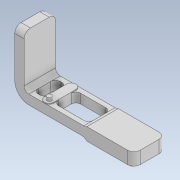
# Autodesk Inventor part: LBody
Saved by Autodesk Inventor 2020 (Build 240168000, 168)
## iProperties
Created: 2020-03-03
Part Number: LBody
Material: Generic
Document SubType Name: Modeling
Designer: Kjell
Density: 1 g/cm^3
Appearance: Default
Author: Kjell
Autodesk Inventor part; units mm, degrees
ref_plane "YZ Plane" through (0, 0, 0) normal (1, 0, 0) x (0, 1, 0)
ref_plane "XZ Plane" through (0, 0, 0) normal (0, 1, 0) x (-1, 0, 0)
ref_plane "XY Plane" through (0, 0, 0) normal (0, 0, 1) x (1, 0, 0)
derived "master_sketch.ipt"
sketch "BottomPlateMainDim" plane through (0, 0, 0) normal (0, 0, 1) x (1, 0, 0)
  circle A0 centre (0, 0) radius 3
  circle A1 centre (-42, -7) radius 1.5
  line L0 (-55, 11) -> (-55, -11)
  line L1 (0, 0) -> (-55, 0)
  line L2 (-15, 10) -> (15, 10)
  line L3 (15, 10) -> (15, -10)
  line L4 (15, -10) -> (-15, -10)
  line L5 (-15, -10) -> (-15, 10)
  line L6 (-15, 10) -> (15, -10) construction
  line L7 (15, 10) -> (-15, -10) construction
sketch "FronProfile" plane through (0, 0, 0) normal (0, 1, 0) x (-1, 0, 0)
  line L0 (-15, 0) -> (-15, 8)
  line L1 (-15, 8) -> (15, 8)
  line L2 (15, 8) -> (15, 0)
  line L3 (15, 7.5) -> (52, 7.5)
  line L4 (15, 1.5) -> (52, 1.5)
  line L5 (15, 0) -> (-15, 0)
  line L6 (55, 10.5) -> (55, 14.7599) construction
  line L7 (55, 10.5) -> (55, 40.5)
  line L8 (55, 40.5) -> (61, 40.5)
  line L9 (61, 40.5) -> (61, 10.5)
  arc A0 (52, 7.5) -> (55, 10.5) centre (52, 10.5) ccw
  arc A1 (52, 1.5) -> (61, 10.5) centre (52, 10.5) ccw
  point P0 (0, 0)
  point P1 (15, 0)
  point P2 (55, 0)
  point P3 (55, 0)
  point P4 (55, 0)
sketch "DovetailWeld" plane through (0, 0, 0) normal (0, 0, 1) x (1, 0, 0)
  line L0 (12, 8) -> (-12, 8)
  line L1 (-12, 8) -> (-12, -8)
  line L2 (-12, -8) -> (12, -8)
  line L3 (12, -8) -> (12, 8)
  line L4 (12, 8) -> (-12, -8) construction
  line L5 (-12, 8) -> (12, -8) construction
  point P0 (0, 0)
extrude "Extrusion1" add sketch "FronProfile" along normal mid plane 20
fillet "Fillet1" radius 4 1 edges at (-15, 0, 7.5)
fillet "Fillet2" radius 4 1 edges at (-15, 0, 1.5)
sketch "Sketch3" plane through (-52, -10, 7.5) normal (0, 0, 1) x (1, 0, 0)
  line L0 (0, 20) -> (35.0635, 20) projected
  circle A0 centre (10, 3) radius 1.5 projected
  line L1 (10, 3) -> (10, 17) construction
  line L2 (13, 3) -> (13, 17)
  line L3 (7, 17) -> (7, 3)
  arc A1 (7, 3) -> (13, 3) centre (10, 3) ccw
  arc A2 (13, 17) -> (7, 17) centre (10, 17) ccw
  point P0 (52, 10)
  point P1 (10, 10)
  dimension "d5" = 6
  constraints: 8 end point, 5 tangent, 4 point on circle, 2 centre point, 1 midpoint, 1 parallel, 1 vertical
  measures "d5" diameter of A2
extrude "Extrusion2" add sketch "Sketch3" along normal blind 2.5 contours A0
extrude "Extrusion3" add sketch "Sketch3" along normal up to surface (0.5 mm away)
sketch "Sketch4" plane through (-16.9365, -10, 7.5) normal (0, 0, 1) x (1, 0, 0)
  line L0 (0, 0) -> (-25.0635, 0) projected
  line L1 (0, 20) -> (0, 0) projected
  line L2 (-25.0635, 20) -> (0, 20) projected
  line L3 (-22.0635, 17) -> (-22.0635, 3) projected
  line L4 (-25.0635, 0) -> (-35.0635, 0) projected
  line L5 (-35.0635, 0) -> (-35.0635, 20) projected
  line L6 (-28.0635, 3) -> (-28.0635, 17) projected
  line L7 (-22.0635, 17) -> (-22.0635, 3) projected
  line L8 (-19.0635, 17) -> (-3, 17)
  line L9 (0, 14) -> (0, 6)
  line L10 (-3, 3) -> (-19.0635, 3)
  line L11 (-22.0635, 6) -> (-22.0635, 14)
  arc A0 (-19.0635, 17) -> (-22.0635, 14) centre (-19.0635, 14) ccw
  arc A1 (0, 14) -> (-3, 17) centre (-3, 14) ccw
  arc A2 (-3, 3) -> (0, 6) centre (-3, 6) ccw
  arc A3 (-22.0635, 6) -> (-19.0635, 3) centre (-19.0635, 6) ccw
  line L12 (-32.0635, 17) -> (-31.0635, 17)
  line L13 (-28.0635, 14) -> (-28.0635, 6)
  line L14 (-31.0635, 3) -> (-32.0635, 3)
  line L15 (-35.0635, 6) -> (-35.0635, 14)
  arc A4 (-32.0635, 17) -> (-35.0635, 14) centre (-32.0635, 14) ccw
  arc A5 (-28.0635, 14) -> (-31.0635, 17) centre (-31.0635, 14) ccw
  arc A6 (-31.0635, 3) -> (-28.0635, 6) centre (-31.0635, 6) ccw
  arc A7 (-35.0635, 6) -> (-32.0635, 3) centre (-32.0635, 6) ccw
  point P0 (16.9365, 10)
  dimension "Wall" = 3
  dimension "d11" = 3
  dimension "d12" = 3
  dimension "d13" = 3
  constraints: 16 end point, 16 point on circle, 16 tangent, 8 centre point, 6 collinear, 6 equal radius, 4 parallel, 2 horizontal, 2 perpendicular
  measures "Wall" distance between parallel lines of L2 L8
  measures "d11" distance between parallel lines of L10 L0
  measures "d12" radius of A0
  measures "d13" radius of A4
extrude "Extrusion4" cut sketch "Sketch4" against normal through all
fillet "Fillet3" radius 4 4 edges at (15, -10, 4) (15, 10, 4) (-58, -10, 40.5) (-58, 10, 40.5)
sketch "Sketch5" plane through (-15, -10, 0) normal (0, 0, -1) x (-1, 0, 0)
  circle A0 centre (-15, 10) radius 6.5
  line L0 (-3, 2) -> (-27, 2) projected
  line L1 (-3, 18) -> (-3, 2) projected
  line L2 (-27, 18) -> (-3, 18) projected
  line L3 (-27, 2) -> (-27, 18) projected
  dimension "d17" = 13
  constraints: 1 centre point, 1 coincident
  measures "d17" diameter of A0
extrude "Extrusion5" cut sketch "Sketch5" against normal blind 3 contours A0
extrude "Extrusion6" add sketch "Sketch5" along normal blind 2
fillet "Fillet4" radius 2 4 edges at (12, 8, -1) (12, -8, -1) (-12, 8, -1) (-12, -8, -1)
offset faces "Size1" outward -0.1 faces at (3.3333, -8, -0.6667) (11.3603, -7.4661, -0.6667) (-11.7321, -7, -0.6667) (-12, -2, -0.6667) (12, 2, -0.6667) (11.3603, 7.4661, -0.6667) (-3.3333, 8, -0.6667) (-11.4661, 7.3603, -0.6667)
equation "\"d11\" = Wall"
body "Solid1"
